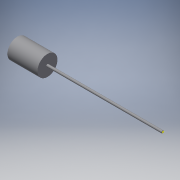
# Autodesk Inventor part: Drill 8
Saved by Autodesk Inventor 2018 (Build 220112000, 112)
## iProperties
Created: 2021-03-25
Part Number: Drill 8
Material: Generic
Document SubType Name: Modeling
Designer: Charles.Rymal
Density: 1 g/cm^3
Appearance: Default
Author: Charles.Rymal
Autodesk Inventor part; units mm, degrees
ref_plane "YZ Plane" through (0, 0, 0) normal (1, 0, 0) x (0, 1, 0)
ref_plane "XZ Plane" through (0, 0, 0) normal (0, 1, 0) x (-1, 0, 0)
ref_plane "XY Plane" through (0, 0, 0) normal (0, 0, 1) x (1, 0, 0)
sketch "Sketch1" plane through (0, 0, 0) normal (0, 0, 1) x (1, 0, 0)
  line L0 (-12.4424, 3.175) -> (279.6576, 3.175)
  line L1 (279.6576, 3.175) -> (279.6576, 0)
  line L2 (279.6576, 0) -> (0, 0)
  line L3 (0, 0) -> (-88.6424, 0)
  line L4 (-88.6424, 0) -> (-88.6424, 25.4)
  line L5 (-88.6424, 25.4) -> (-12.4424, 25.4)
  line L6 (-12.4424, 25.4) -> (-12.4424, 3.175)
  dimension "d0" = 3.175
  dimension "d1" = 292.1
  dimension "d2" = 25.4
  dimension "d3" = 76.2
  constraints: 15 end point, 5 perpendicular, 1 horizontal, 1 point on line
  measures "d0" distance between parallel lines of L2 L0
  measures "d1" distance of L0.start L0.end
  measures "d2" distance between parallel lines of L3 L5
  measures "d3" distance of L4.end L5.end
revolve "Revolution1" add sketch "Sketch1" angle 360 about axis through (0, 0, 0) along (-1, 0, 0)
body "Solid1"
